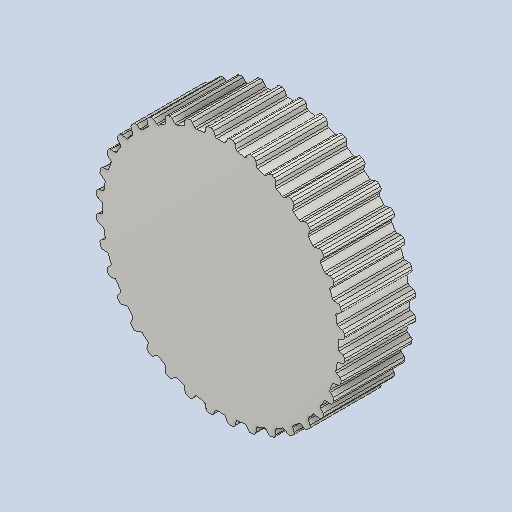
# Autodesk Inventor part: Synchronous Pulley2
Saved by Autodesk Inventor 2022.2 (Build 262287000, 287)
## iProperties
Created: 2022-01-08
Part Number: Synchronous Pulley2
Material: Steel
Document SubType Name: Modeling
Designer: Jochen
Density: 1 g/cm^3
Appearance: Steel
CustomPartVersion: 1
Author: Jochen
Autodesk Inventor part; units mm, degrees
ref_plane "YZ Plane" through (0, 0, 0) normal (1, 0, 0) x (0, 1, 0)
ref_plane "XZ Plane" through (0, 0, 0) normal (0, 1, 0) x (-1, 0, 0)
ref_plane "XY Plane" through (0, 0, 0) normal (0, 0, 1) x (1, 0, 0)
sketch "Pulley Sketch" plane through (0, 0, 0) normal (0, 0, 1) x (1, 0, 0)
  circle A0 centre (0, 0) radius 14.3239 construction
  circle A1 centre (0, 0) radius 14.0239
  circle A2 centre (0, 0) radius 13.2739
  line L0 (-0.8624, 13.9974) -> (-0.525, 13.2739)
  line L1 (-0.525, 13.2739) -> (0.525, 13.2739)
  line L2 (0.525, 13.2739) -> (0.8624, 13.9974)
  line L3 (0, 0) -> (0, 14.0239) construction
  point P0 (0, 13.2739)
  dimension "d0" = 28.6479
  dimension "d1" = 0.3
  dimension "d2" = 0.75
  dimension "d3" = 50
  dimension "d4" = 1.05
  constraints: 8 end point, 3 coincident, 3 point on circle, 2 centre point, 1 horizontal, 1 midpoint, 1 point on line, 1 vertical, 1 vertical alignment, 3 other
  measures "d0" diameter of A0
  measures "d1" radial gap between concentric circles of A0 A1
  measures "d3" angle of L2 L0
  measures "d4" distance of L0.end L1.end
extrude "Base Body" add sketch "Pulley Sketch" along normal mid plane 8 contours A2 | A1 L0 L1 L2 | L2 L1 L0 A1
extrude "Tooth" cut sketch "Pulley Sketch" along normal through all both and the other way through all contours L2 L1 L0 A1 picked at (0, 13.7719)
fillet "Tooth Fillet" radius 0.2 2 edges at (0.525, 13.2739, 0) (-0.525, 13.2739, 0)
fillet "Tooth Fillet" radius 0.3 4 edges at (-0.8624, 13.9974, 2) (-0.8624, 13.9974, -2) (0.8624, 13.9974, 2) (0.8624, 13.9974, -2)
pattern_circular "Teeth" count 36 over 360 about axis through (0, 0, -10) along (0, 0, 1) of "Tooth", "Tooth Fillet"
feature "Left flange" [suppressed]
feature "Right flange" [suppressed]
equation "\"d1\" = da_a"
equation "\"d2\" = da_hg"
equation "\"d3\" = 2 * da_fi"
equation "\"d4\" = da_bw"
equation "\"d5\" = da_bf"
equation "\"d7\" = da_bf"
equation "\"d9\" = da_rb"
equation "\"d10\" = da_rt"
equation "\"da_pb\" = 2.5"
equation "\"da_fi\" = 25deg"
equation "\"da_hg\" = 0.75"
equation "\"da_bw\" = 1.05"
equation "\"da_rb\" = 0.2"
equation "\"da_rt\" = 0.3"
equation "\"da_a\" = 0.3"
equation "\"da_bf\" = 8"
equation "\"da_wf\" = 1.5"
equation "\"da_hf\" = 1.5"
body "Solid1"
